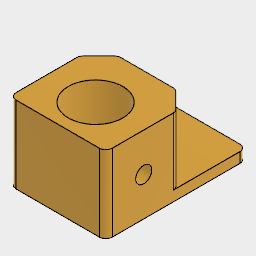
Y_End_Stop_Flag_F01 (Autodesk Fusion 360 design; units mm, degrees)
Autodesk Fusion 360 part; units mm, degrees
sketch "スケッチ1" plane through (0, 0, 0) normal (0, 0, 1) x (1, 0, 0)
  line L0 (7.5, 16) -> (-7.5, 16)
  line L1 (-7.5, 16) -> (-7.5, -5.9)
  line L2 (-7.5, -5.9) -> (7.5, -5.9)
  line L3 (7.5, -5.9) -> (7.5, 16)
  line L4 (7.5, 16) -> (-7.5, -5.9) construction
  line L5 (-7.5, 16) -> (7.5, -5.9) construction
  circle A0 centre (0, 0) radius 4.25
  line L6 (-7.5, 5) -> (-4.5, 8)
  line L7 (-4.5, 8) -> (4.5, 8)
  line L8 (4.5, 8) -> (7.5, 5)
  point P0 (0, 5.05)
  dimension "d1" = 15
  dimension "d2" = 21.9
  dimension "d3" = 8.5
  dimension "d4" = 5.9
  dimension "d5" = 13.9
  dimension "d6" = 45
  dimension "d7" = 45
  dimension "d8" = 3
  dimension "d9" = 3
  measures "d1" distance of L1.end L2.end
  measures "d2" distance of L0.end L1.end
  measures "d3" diameter of A0
  measures "d4" distance of A0.centre L2
  measures "d5" distance of L2 L7
  measures "d6" angle of L3 L8
  measures "d7" angle of L1 L6
  measures "d8" distance of L1 L6.end
  measures "d9" distance of L3 L7.end
extrude "押し出し1" add sketch "スケッチ1" along normal blind 12 contours L1 L2 L3 L6 L7 L8
extrude "押し出し2" add sketch "スケッチ1" along normal blind 1.6 contours L0 L1 L3 L6 L7 L8
hole "穴1" at (7.5, 0, 6) direction (-1, 0, 0) diameter 2.5 depth 16 tip angle 118
fillet "フィレット1" radius 1 8 edges at (-7.5, -5.9, 6) (7.5, -5.9, 6) (7.5, 5, 6.8) (4.5, 8, 6.8) (-4.5, 8, 6.8) (-7.5, 5, 6.8) (-7.5, 16, 0.8) (7.5, 16, 0.8)
